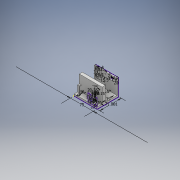
# Autodesk Inventor part: pnp-head
Saved by Autodesk Inventor 2017 (Build 210142000, 142)
## iProperties
Created: 2026-03-22
Part Number: pnp-head
Material: Generic
Document SubType Name: Modeling
Designer: a
Density: 1 g/cm^3
Appearance: Default
Author: a
Autodesk Inventor part; units mm, degrees
note: some values were not read from the file. Chosen so that the rebuilt part matches the saved one: sketch regions of "Extrusion1".
ref_plane "YZ Plane" through (0, 0, 0) normal (1, 0, 0) x (0, 1, 0)
ref_plane "XZ Plane" through (0, 0, 0) normal (0, 1, 0) x (-1, 0, 0)
ref_plane "XY Plane" through (0, 0, 0) normal (0, 0, 1) x (1, 0, 0)
sketch "Sketch1" plane through (0, 0, 0) normal (0, 0, 1) x (1, 0, 0)
  line L0 (0, 0) -> (75, 0)
  line L1 (75, 0) -> (75, -71.001)
  line L2 (75, -71.001) -> (0, -71.001)
  line L3 (0, -71.001) -> (0, 0)
  circle A0 centre (15, -29) radius 2.5
  circle A1 centre (25, -29) radius 2.5
  circle A2 centre (35, -29) radius 2.5
  circle A3 centre (25, -19) radius 2.5
  circle A4 centre (25, -39) radius 2.5
  circle A5 centre (4.85, -29) radius 2.5
  circle A6 centre (4.85, -39) radius 2.5
  circle A7 centre (4.85, -19) radius 2.5
  circle A8 centre (45.15, -19) radius 2.5
  circle A9 centre (45.15, -39) radius 2.5
  line L4 (0, 0) -> (50, 0)
  line L5 (50, 0) -> (50, -5)
  line L6 (0, -5) -> (0, 0)
  line L7 (0, -5) -> (75, -5)
  line L8 (0, -44) -> (75, -44)
  line L9 (0, -54) -> (75, -54)
  line L10 (0, -68) -> (75, -68)
  line L11 (0, -71) -> (75, -71)
  line L12 (45, -68) -> (45, -71)
  line L13 (6, -54) -> (6, -68)
  line L14 (0, -57) -> (6, -57)
  line L15 (0, -60) -> (6, -60)
  point P0 (37.5, 0)
  dimension "d0" = 75
  dimension "d1" = 71.001
  dimension "d3" = 5
  dimension "d4" = 10
  dimension "d6" = 10
  dimension "d8" = 10
  dimension "d10" = 10
  dimension "d12" = 20.15
  dimension "d15" = 20.15
  dimension "d23" = 5
  dimension "d29" = 39
  dimension "d30" = 15
  dimension "d31" = 10
  dimension "d44" = 14
  dimension "d45" = 3
  dimension "d46" = 25
  dimension "d52" = 30
  dimension "d69" = 6
  dimension "d71" = 3
  dimension "d72" = 3
  constraints: 30 end point, 11 point on line, 10 centre point, 9 equal radius, 9 perpendicular, 7 horizontal alignment, 5 vertical alignment, 4 horizontal, 2 parallel, 1 midpoint, 1 vertical, 10 other
  measures "d0" distance of L1.end L2.end
  measures "d1" distance of L0.end L1.end
  measures "d3" diameter of A1
  measures "d4" distance of A0.centre A1.centre
  measures "d6" distance of A1.centre A2.centre
  measures "d8" distance of A1.centre A3.centre
  measures "d10" distance of A4.centre A1.centre
  measures "d12" distance of A1.centre A5.centre
  measures "d15" horizontal distance of A1.centre A8.centre
  measures "d23" distance between parallel lines of L0 L7
  measures "d29" distance between parallel lines of L7 L8
  measures "d30" distance from line of L8 A1.centre
  measures "d31" distance between parallel lines of L8 L9
  measures "d44" distance between parallel lines of L9 L10
  measures "d45" distance between parallel lines of L10 L11
  measures "d52" distance between parallel lines of L1 L12
  measures "d69" distance of the line from the sketch origin of L13
  measures "d71" distance between parallel lines of L9 L14
  measures "d72" distance between parallel lines of L14 L15
sketch "Sketch1 outline for Extrusion1" plane through (0, 0, 0) normal (0, 0, 1) x (1, 0, 0)
  line L0 (75, 0) -> (0, 0)
  line L1 (0, 0) -> (0, -71.001)
  line L2 (0, -71.001) -> (75, -71.001)
  line L3 (75, -71.001) -> (75, 0)
  circle A0 centre (45.15, -19) radius 2.5
  circle A1 centre (4.85, -39) radius 2.5
  circle A2 centre (45.15, -39) radius 2.5
  circle A3 centre (4.85, -19) radius 2.5
extrude "Extrusion1" add sketch "Sketch1 outline for Extrusion1" along normal blind 6
sketch "Sketch1 outline for Extrusion3" plane through (0, 0, 0) normal (0, 0, 1) x (1, 0, 0)
  line L0 (75, 0) -> (0, 0)
  line L1 (75, -5) -> (75, 0)
  line L2 (0, -5) -> (75, -5)
  line L3 (0, 0) -> (0, -5)
  line L4 (75, -44) -> (0, -44)
  line L5 (75, -54) -> (75, -44)
  line L6 (0, -54) -> (75, -54)
  line L7 (0, -44) -> (0, -54)
extrude "Extrusion3" add sketch "Sketch1 outline for Extrusion3" along normal blind 54
sketch "Sketch3" plane through (0, 0, 0) normal (0, 1, 0) x (1, 0, 0)
  line L0 (0, -54) -> (75, -54) projected
  line L1 (0, 0) -> (75, 0)
  line L2 (75, 0) -> (75, -54)
  line L3 (75, -54) -> (0, -54)
  line L4 (0, -54) -> (0, 0)
  circle A0 centre (5.5, -48.5) radius 1.65
  circle A1 centre (36.5, -48.5) radius 1.65
  circle A2 centre (5.5, -17.5) radius 1.65
  circle A3 centre (36.5, -17.5) radius 1.65
  line L5 (21, -33) -> (21, -54) construction
  line L6 (18.4, -33) -> (18.4, -54)
  line L7 (23.6, -54) -> (23.6, -33)
  arc A4 (23.6, -33) -> (18.4, -33) centre (21, -33) ccw
  arc A5 (18.4, -54) -> (23.6, -54) centre (21, -54) ccw
  circle A6 centre (55, -44) radius 5
  point P0 (21, -43.5)
  dimension "d34" = 3.3
  dimension "d35" = 31
  dimension "d36" = 31
  dimension "d37" = 5.2
  dimension "d38" = 15.5
  dimension "d39" = 15.5
  dimension "d40" = 21
  dimension "d41" = 21
  dimension "d47" = 10
  dimension "d48" = 10
  dimension "d49" = 20
  constraints: 16 end point, 7 centre point, 4 point on circle, 4 tangent, 3 equal radius, 3 parallel, 2 horizontal alignment, 2 perpendicular, 2 vertical alignment, 1 horizontal, 1 midpoint, 1 point on line
  measures "d34" diameter of A0
  measures "d35" distance of A0.centre A2.centre
  measures "d36" distance of A1.centre A0.centre
  measures "d37" diameter of A5
  measures "d38" horizontal distance of A0.centre L5.start
  measures "d39" horizontal distance of A2.centre L5.start
  measures "d40" distance from line of L3 L5.start
  measures "d41" distance from line of L4 L5.start
  measures "d47" diameter of A6
  measures "d48" distance from line of L3 A6.centre
  measures "d49" distance from line of L2 A6.centre
sketch "Sketch3 outline for Extrusion5" plane through (0, 0, 0) normal (0, 1, 0) x (1, 0, 0)
  arc A0 (23.6, -33) -> (18.4, -33) centre (21, -33) ccw
  line L0 (23.6, -54) -> (23.6, -33)
  arc A1 (18.4, -54) -> (23.6, -54) centre (21, -54) ccw
  line L1 (18.4, -33) -> (18.4, -54)
  circle A2 centre (5.5, -48.5) radius 1.65
  circle A3 centre (36.5, -48.5) radius 1.65
  circle A4 centre (5.5, -17.5) radius 1.65
  circle A5 centre (36.5, -17.5) radius 1.65
extrude "Extrusion5" cut sketch "Sketch3 outline for Extrusion5" against normal blind 5
sketch "Sketch3 outline for Extrusion6" plane through (0, 0, 0) normal (0, 1, 0) x (1, 0, 0)
  circle A0 centre (55, -44) radius 5
extrude "Extrusion6" cut sketch "Sketch3 outline for Extrusion6" against normal blind 54
sketch "Sketch1 outline for Extrusion7" plane through (0, 0, 0) normal (0, 0, 1) x (1, 0, 0)
  line L0 (75, -71) -> (75, -68)
  line L1 (45, -71) -> (75, -71)
  line L2 (45, -68) -> (45, -71)
  line L3 (75, -68) -> (45, -68)
extrude "Extrusion7" add sketch "Sketch1 outline for Extrusion7" along normal blind 32
sketch "Sketch4" plane through (45, -71, 6) normal (0, -1, 0) x (1, 0, 0)
  line L0 (0, 0) -> (30, 0) projected
  line L1 (0, 26) -> (30, 26) projected
  line L2 (0, 0) -> (30, 0)
  line L3 (30, 0) -> (30, 26)
  line L4 (30, 26) -> (0, 26)
  line L5 (0, 26) -> (0, 0)
  circle A0 centre (22.5, 24) radius 1
  circle A1 centre (22.5, 3) radius 1
  circle A2 centre (10, 3) radius 1
  circle A3 centre (10, 24) radius 1
  line L6 (0, 0) -> (0, 26) projected
  line L7 (15.5, 8) -> (4.5, 8)
  line L8 (4.5, 8) -> (4.5, 19)
  line L9 (4.5, 19) -> (15.5, 19)
  line L10 (15.5, 19) -> (15.5, 8)
  line L11 (15.5, 8) -> (4.5, 19) construction
  line L12 (4.5, 8) -> (15.5, 19) construction
  point P0 (-45, -6)
  point P1 (10, 13.5)
  point P2 (10, 13.5)
  point P3 (10, 13.5)
  dimension "d55" = 2
  dimension "d58" = 12.5
  dimension "d59" = 21
  dimension "d60" = 2
  dimension "d61" = 11
  dimension "d62" = 11
  dimension "d63" = 10.5
  dimension "d68" = 20
  constraints: 20 end point, 4 centre point, 4 midpoint, 4 parallel, 3 equal radius, 3 vertical alignment, 2 horizontal, 2 horizontal alignment, 2 perpendicular
  measures "d55" diameter of A0
  measures "d58" distance of A0.centre A3.centre
  measures "d59" distance of A1.centre A0.centre
  measures "d60" distance from line of L1 A0.centre
  measures "d61" distance of L8.end L9.end
  measures "d62" distance of L7.end L8.end
  measures "d63" distance of A2.centre point (10, 13.5)
  measures "d68" distance from line of L3 point (10, 13.5)
sketch "Sketch4 outline for Extrusion8" plane through (45, -71, 6) normal (0, -1, 0) x (1, 0, 0)
  line L0 (15.5, 8) -> (4.5, 8)
  line L1 (4.5, 8) -> (4.5, 19)
  line L2 (4.5, 19) -> (15.5, 19)
  line L3 (15.5, 19) -> (15.5, 8)
extrude "Extrusion8" cut sketch "Sketch4 outline for Extrusion8" against normal blind 3
sketch "Sketch4 outline for Extrusion9" plane through (45, -71, 6) normal (0, -1, 0) x (1, 0, 0)
  circle A0 centre (22.5, 24) radius 1
  circle A1 centre (22.5, 3) radius 1
  circle A2 centre (10, 3) radius 1
  circle A3 centre (10, 24) radius 1
extrude "Extrusion9" add sketch "Sketch4 outline for Extrusion9" against normal blind 6
sketch "Sketch1 outline for Extrusion10" plane through (0, 0, 0) normal (0, 0, 1) x (1, 0, 0)
  line L0 (6, -57) -> (0, -57)
  line L1 (6, -60) -> (6, -57)
  line L2 (0, -60) -> (6, -60)
  line L3 (0, -57) -> (0, -60)
extrude "Extrusion10" add sketch "Sketch1 outline for Extrusion10" along normal blind 26
sketch "Sketch5" plane through (0, -60, 6) normal (0, -1, 0) x (1, 0, 0)
  line L0 (6, 20) -> (0, 20)
  line L1 (0, -1.548307) -> (6, -1.548307)
  line L2 (6, -1.548307) -> (6, 20)
  line L3 (6, 20) -> (0, 20)
  line L4 (0, 20) -> (0, -1.548307)
  line L5 (0, 17) -> (6, 17)
  point P0 (0, -6)
  dimension "d75" = 3
  constraints: 10 end point, 2 horizontal, 2 parallel, 2 point on line, 1 perpendicular
  measures "d75" distance between parallel lines of L0 L5
sketch "Sketch5 outline for Extrusion11" plane through (0, -60, 6) normal (0, -1, 0) x (1, 0, 0)
  line L0 (6, 17) -> (6, 20)
  line L1 (0, 17) -> (6, 17)
  line L2 (0, 20) -> (0, 17)
  line L3 (6, 20) -> (0, 20)
extrude "Extrusion11" add sketch "Sketch5 outline for Extrusion11" against normal blind 6
fillet "Fillet1" radius 0.75 7 edges at (6, -57, 14.5) (0, -57, 14.5) (0, -54, 14.5) (0, -55.5, 23) (0, -55.5, 6) (6, -55.5, 23) (45, -68, 19)
body "Solid1"
